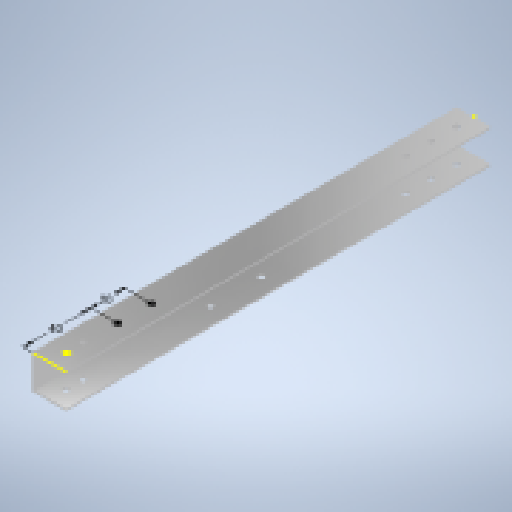
# Autodesk Inventor part: gear_plate_pole
Saved by Autodesk Inventor 2024.1 (Build 281209000, 209)
## iProperties
Created: 2025-09-25
Part Number: gear_plate_pole
Material: アルミニウム 6061
Document SubType Name: Modeling
Designer: hibik
Density: 2.7 g/cm^3
Appearance: アルミニウム - フラット
Author: hibik
Autodesk Inventor part; units mm, degrees
ref_plane "YZ Plane" through (0, 0, 0) normal (1, 0, 0) x (0, 1, 0)
ref_plane "XZ Plane" through (0, 0, 0) normal (0, 1, 0) x (-1, 0, 0)
ref_plane "XY Plane" through (0, 0, 0) normal (0, 0, 1) x (1, 0, 0)
sketch "スケッチ1" plane through (0, 0, 0) normal (0, 0, 1) x (1, 0, 0)
  line L0 (-10, -10) -> (10, -10)
  line L1 (10, -10) -> (10, 10)
  line L2 (10, 10) -> (-10, 10)
  line L3 (-10, 10) -> (-10, -10)
  line L4 (-10, -10) -> (10, 10) construction
  line L5 (10, -10) -> (-10, 10) construction
  line L6 (9, -9) -> (-9, -9)
  line L7 (-9, -9) -> (-9, 9)
  line L8 (-9, 9) -> (9, 9)
  line L9 (9, 9) -> (9, -9)
  line L10 (9, -9) -> (-9, 9) construction
  line L11 (-9, -9) -> (9, 9) construction
  line L12 (9, 9) -> (10, 9)
  line L13 (9, -9) -> (10, -9)
  point P0 (0, 0)
  dimension "d0" = 20
  dimension "d1" = 20
  dimension "d2" = 1
  constraints: 28 end point, 4 midpoint, 4 parallel, 4 perpendicular, 3 point on line, 2 horizontal
  measures "d0" distance of L2.end L1.end
  measures "d1" distance of L1.end L0.end
  measures "d2" distance between parallel lines of L2 L8
extrude "押し出し1" add sketch "スケッチ1" along normal blind 250 contours L3 L2 L1 L12 L8 L7 L6 L13 L0
sketch "スケッチ2" plane through (-10, -10, 0) normal (0, -1, 0) x (1, 0, 0)
  circle A0 centre (10, 155) radius 1.75
  circle A1 centre (10, 125) radius 1.75
  line L0 (0, 0) -> (0, 250) projected
  line L1 (0, 250) -> (20, 250) projected
  point P0 (10, 0)
  dimension "d5" = 3.5
  dimension "d7" = 10
  dimension "d8" = 95
  dimension "d9" = 30
  constraints: 2 centre point, 1 equal radius, 1 vertical alignment
  measures "d5" diameter of A0
  measures "d7" distance from line of L0 A0.centre
  measures "d8" distance from line of L1 A0.centre
  measures "d9" distance of A0.centre A1.centre
extrude "押し出し2" cut sketch "スケッチ2" against normal up to surface (1 mm away)
sketch "スケッチ3" plane through (-9, -9, 0) normal (1, 0, 0) x (0, 0, -1)
  line L0 (-156.75, 0) -> (-153.25, 0) projected
  circle A0 centre (-170, 9) radius 2.25
  circle A1 centre (-140, 9) radius 2.25
  line L1 (0, -1) -> (-250, -1) projected
  point P0 (0, 9)
  point P1 (-155, 0)
  dimension "d12" = 4.5
  dimension "d13" = 4.5
  dimension "d14" = 15
  dimension "d15" = 10
  dimension "d16" = 30
  constraints: 2 centre point, 1 horizontal alignment, 1 midpoint
  measures "d12" diameter of A0
  measures "d13" diameter of A1
  measures "d14" horizontal distance of A0.centre point (-155, 0)
  measures "d15" distance from line of L1 A0.centre
  measures "d16" distance of A1.centre A0.centre
extrude "押し出し3" cut sketch "スケッチ3" against normal through all
sketch "スケッチ5" plane through (-10, 10, 0) normal (0, 1, 0) x (1, 0, 0)
  circle A0 centre (10, -240) radius 1.75
  circle A1 centre (10, -10) radius 1.75
  circle A2 centre (10, -25) radius 1.75
  circle A3 centre (10, -230) radius 1.75
  circle A4 centre (10, -40) radius 1.75
  line L0 (20, 0) -> (0, 0) projected
  line L1 (20, -250) -> (0, -250) projected
  point P0 (10, 0)
  point P1 (10, 0)
  dimension "d19" = 3.5
  dimension "d20" = 10
  dimension "d21" = 10
  dimension "d22" = 10
  dimension "d23" = 15
  dimension "d24" = 15
  constraints: 5 centre point, 5 vertical alignment, 4 equal radius, 1 midpoint
  measures "d19" diameter of A0
  measures "d20" distance from line of L1 A0.centre
  measures "d21" distance of A0.centre A3.centre
  measures "d22" distance from line of L0 A1.centre
  measures "d23" distance of A2.centre A1.centre
  measures "d24" distance of A4.centre A2.centre
extrude "押し出し4" cut sketch "スケッチ5" against normal through all
sketch "スケッチ6" plane through (-10, 10, 0) normal (0, 1, 0) x (1, 0, 0)
  circle A0 centre (10, -210) radius 1.75
  circle A1 centre (10, -190) radius 1.75
  circle A2 centre (10, -240) radius 1.75 projected
  line L0 (20, -250) -> (0, -250) projected
  point P0 (10, 0)
  dimension "d27" = 40
  dimension "d28" = 20
  constraints: 2 centre point, 2 equal radius, 2 vertical alignment
  measures "d27" distance from line of L0 A0.centre
  measures "d28" distance of A0.centre A1.centre
extrude "押し出し5" cut sketch "スケッチ6" against normal through all contours A0 | A1
equation "\"d24\" = d23"
